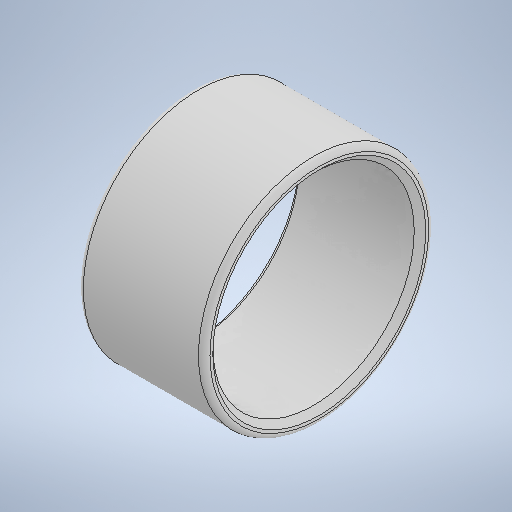
# Autodesk Inventor part: 26-10-203
Saved by Autodesk Inventor 2025.2 (Build 292293000, 293)
## iProperties
Created: 2024-11-29
Part Number: 26-10-203
Material: Generic
Document SubType Name: Modeling
Designer: Zvonko.Gabric
Density: 1 g/cm^3
Appearance: Default
Description: Tensioning wheel Stage 1, Belt tensioner
Author: Zvonko.Gabric
Autodesk Inventor part; units mm, degrees
ref_plane "YZ Plane" through (0, 0, 0) normal (1, 0, 0) x (0, 1, 0)
ref_plane "XZ Plane" through (0, 0, 0) normal (0, 1, 0) x (-1, 0, 0)
ref_plane "XY Plane" through (0, 0, 0) normal (0, 0, 1) x (1, 0, 0)
sketch "Sketch1" plane through (0, 0, 0) normal (0, 1, 0) x (-1, 0, 0)
  line L0 (20, -1.5) -> (21, -0.5)
  line L1 (0, -1.5) -> (20, -1.5)
  line L2 (-1, -0.5) -> (0, -1.5)
  line L3 (-1, 0) -> (-1, -0.5)
  line L4 (20, 1) -> (0, 1)
  line L5 (21, -0.5) -> (21, 0)
  arc A0 (0, 1) -> (-1, 0) centre (0, 0) ccw
  arc A1 (21, 0) -> (20, 1) centre (20, 0) ccw
  line L6 (20, -19) -> (-1, -19) construction
  dimension "d0" = 0
  dimension "d1" = 20
  dimension "d2" = 1.4142
  dimension "d3" = 135
  dimension "d4" = 2.5
  dimension "d5" = 1
  dimension "d6" = 1.5
  dimension "d7" = 20
  dimension "d8" = 22
  dimension "d9" = 1
  dimension "d10" = 1.5
  dimension "d11" = 1
  dimension "d12" = 1
  dimension "d13" = 135
  dimension "d14" = 90
  dimension "d15" = 90
  dimension "d16" = 17.5
  constraints: 14 end point, 4 point on circle, 2 centre point, 1 horizontal
  measures "d0" distance of point (0, 0) A0.centre
  measures "d1" distance of L1.start L0.start
  measures "d2" distance of L0.start L0.end
  measures "d3" angle of L0 L1
  measures "d4" distance between parallel lines of L4 L1
  measures "d5" radius of A1
  measures "d6" distance from line of L1 A1.centre
  measures "d7" distance of L4.start L4.end
  measures "d8" distance of L3.start L5.end
  measures "d9" radius of A0
  measures "d10" distance from line of L1 point (0, 0)
  measures "d11" distance from line of L3 point (0, 0)
  measures "d12" distance from line of L5 A1.centre
  measures "d13" angle of L1 L2
  measures "d14" angle of L4 L3
  measures "d15" angle of L5 L4
  measures "d16" distance between parallel lines of L6 L1
revolve "Revolution1" add sketch "Sketch1" angle 360 about axis through (-20, 0, -19) along (1, 0, 0)
body "Solid1"
